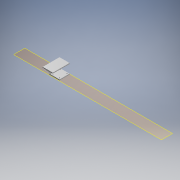
# Autodesk Inventor part: X-portal-column
Saved by Autodesk Inventor 2016 (Build 200138000, 138)
## iProperties
Created: 2015-05-03
Part Number: X-portal-column
Material: Aluminum 6061
Document SubType Name: Modeling
Designer: ax
Mass: 182.25 g
Surface Area: 295.832 cm^2
Volume: 67.5 cm^3
Density: 2.7 g/cm^3
Appearance: Aluminum - Flat
Author: ax
Autodesk Inventor part; units mm, degrees
ref_plane "YZ Plane" through (0, 0, 0) normal (1, 0, 0) x (0, 1, 0)
ref_plane "XZ Plane" through (0, 0, 0) normal (0, 1, 0) x (-1, 0, 0)
ref_plane "XY Plane" through (0, 0, 0) normal (0, 0, 1) x (1, 0, 0)
ref_plane "Work Plane1" through (-170, -5, 0) normal (0, 0, 1) x (1, 0, 0)
sketch "Sketch1" plane through (-170, -5, 0) normal (0, 0, 1) x (1, 0, 0)
  line L0 (170, 5) -> (230, 5)
  line L1 (230, 5) -> (230, -95)
  line L2 (230, -95) -> (170, -95)
  line L3 (170, -95) -> (170, 5)
  dimension "d0" = 60
  dimension "d1" = 100
  constraints: 8 end point, 2 parallel, 1 horizontal, 1 perpendicular
  measures "d0" distance of L1.end L2.end
  measures "d1" distance of L0.end L1.end
extrude "Extrusion1" add sketch "Sketch1" along normal blind 5
sketch "Sketch2" plane through (-170, -5, 5) normal (0, 0, 1) x (1, 0, 0)
  line L0 (170, -95) -> (230, -95) projected
  line L1 (170, 5) -> (175, 5)
  line L2 (175, 5) -> (175, -95)
  line L3 (175, -95) -> (170, -95)
  line L4 (170, -95) -> (170, 5)
  dimension "d4" = 5
  constraints: 8 end point, 2 parallel, 1 horizontal, 1 perpendicular, 1 point on line
  measures "d4" distance of L2.end L3.end
extrude "Extrusion2" add sketch "Sketch2" along normal blind 50
sketch "Sketch3" plane through (-170, -5, 55) normal (0, 0, 1) x (1, 0, 0)
  line L0 (170, -95) -> (170, 5) projected
  line L1 (230, -95) -> (170, -95) projected
  line L2 (170, 5) -> (230, 5)
  line L3 (230, 5) -> (230, -95)
  line L4 (230, -95) -> (170, -95)
  line L5 (170, -95) -> (170, 5)
  dimension "d7" = 60
  constraints: 8 end point, 2 parallel, 1 horizontal, 1 perpendicular
  measures "d7" distance of L1.start L4.end
extrude "Extrusion3" add sketch "Sketch3" along normal blind 5
sketch "Sketch6" plane through (0, -100, 60) normal (-1, 0, 0) x (0, 0, 1)
  line L0 (-60, 0) -> (0, 0)
  line L1 (-55, 0) -> (-5, 0)
  line L2 (-5, 0) -> (-55, 0)
  line L3 (-55, 100) -> (-55, 40)
  line L4 (-55, 0) -> (-55, 40)
  line L5 (-5, 0) -> (-5, 100) projected
  line L6 (-5, 0) -> (0, 0)
  line L7 (-55, 40) -> (-5, 0)
  point P0 (-60, 100)
  constraints: 14 end point, 1 collinear, 1 horizontal, 1 parallel, 1 point on line
extrude "Extrusion5" cut sketch "Sketch6" against normal blind 5
sketch "Sketch9" plane through (-170, -5, 0) normal (0, 0, -1) x (-1, 0, 0)
  line L0 (0, -55) -> (-800, -55)
  line L1 (-800, -55) -> (-800, 5)
  line L2 (-800, 5) -> (0, 5)
  line L3 (0, 5) -> (0, -55)
  line L4 (-230, -95) -> (-230, 5) projected
  line L5 (-170, -95) -> (-170, 5) projected
  line L6 (-230, -95) -> (-170, -95)
  line L7 (-170, -95) -> (-170, -55)
  line L8 (-170, -55) -> (-230, -55)
  line L9 (-230, -55) -> (-230, -95)
  constraints: 16 end point, 3 horizontal, 2 parallel, 2 point on line, 2 vertical, 1 perpendicular, 4 other
extrude "Extrusion6" cut sketch "Sketch9" against normal blind 5 contours L5 L6 L4 L0
sketch "Sketch10" plane through (-170, -5, 5) normal (0, 0, 1) x (1, 0, 0)
  line L0 (230, -55) -> (230, 5) projected
  line L1 (230, 5) -> (175, 5) projected
  point P0 (170, 5)
  point P1 (222, -3)
  point P2 (222, -47)
  point P3 (183, -3)
  point P4 (183, -47)
  dimension "d17" = 8
  dimension "d18" = 8
  dimension "d21" = 44
  dimension "d24" = 39
  constraints: 1 horizontal, 1 vertical, 3 other
  measures "d17" distance from line of L0 point (222, -3)
  measures "d18" distance from line of L1 point (222, -3)
  measures "d21" distance of point (222, -3) point (222, -47)
  measures "d24" distance of point (222, -3) point (183, -3)
hole "Hole1" at (13, -8, 5) at (13, -52, 5) at (52, -52, 5) at (52, -8, 5) direction (0, 0, -1) diameter 4.134 end through all thread size "M5x0.8" class "6H" standard "ISO Metric profile"
sketch "Sketch11" plane through (5, 0, 55) normal (1, 0, 0) x (0, 0, -1)
  line L0 (50, 0) -> (0, 0) construction
  line L1 (0, -100) -> (0, 0) construction
  point P0 (55, 0)
  point P1 (25, -30)
  point P2 (42, -30)
  point P3 (0, -96.3636)
  dimension "d34" = 30
  dimension "d35" = 25
  dimension "d36" = 17
  dimension "d37" = 30
  measures "d34" distance from line of L0 point (25, -30)
  measures "d35" distance from line of L1 point (25, -30)
  measures "d36" distance of point (25, -30) point (42, -30)
  measures "d37" distance from line of L0 point (42, -30)
hole "Hole2" at (5, -30, 13) at (5, -30, 30) direction (-1, 0, 0) diameter 5 end through all
body "Solid1"
